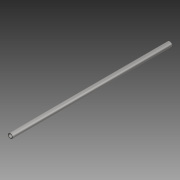
# Autodesk Inventor part: gleitstange
Saved by Autodesk Inventor 2013 (Build 170138000, 138)
## iProperties
Created: 2012-10-19
Part Number: gleitstange
Material: Edelstahl
Document SubType Name: Modeling
Designer: fivef
Density: 8.08 g/cm^3
Mass: 201.55 g
Surface Area: 250.699 cm^2
Volume: 24.9442 cm^3
Author: fivef
Autodesk Inventor part; units mm, degrees
ref_plane "YZ Plane" through (0, 0, 0) normal (1, 0, 0) x (0, 1, 0)
ref_plane "XZ Plane" through (0, 0, 0) normal (0, 1, 0) x (-1, 0, 0)
ref_plane "Arbeitsebene5" through (-13.5, -397, -20) normal (0, 1, 0) x (0, 0, 1)
sketch "Skizze1" plane through (0, 0, 0) normal (0, 1, 0) x (-1, 0, 0)
  circle A0 centre (0, 0) radius 6
  circle A1 centre (0, 0) radius 4
  dimension "d0" = 2
  dimension "d2" = 12
  dimension "d20" = 8
  constraints: 2 centre point, 2 coincident
  measures "d0" radial gap between concentric circles of A0 A1
  measures "d2" diameter of A0
  measures "d20" diameter of A1
extrude "Extrusion1" add sketch "Skizze1" against normal up to surface (397 mm away)
